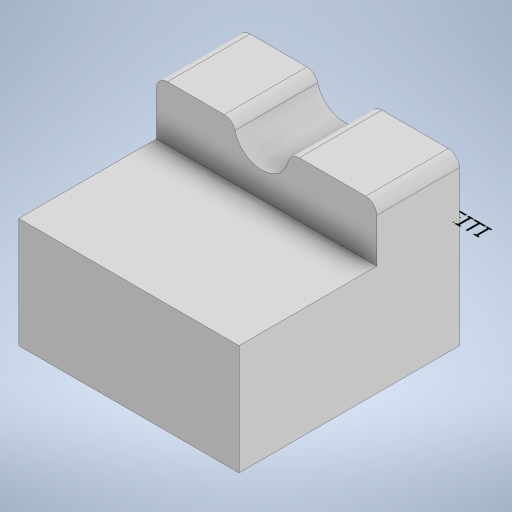
# Autodesk Inventor part: DIODA
Saved by Autodesk Inventor 2023 (Build 270158000, 158)
## iProperties
Created: 2022-12-21
Part Number: DIODA
Material: Generic
Document SubType Name: Sheet Metal
Designer: julia
Density: 1 g/cm^3
Sheet Metal Rule: Default
Appearance: Default
Author: julia
Autodesk Inventor part; units mm, degrees
ref_plane "YZ Plane" through (0, 0, 0) normal (1, 0, 0) x (0, 1, 0)
ref_plane "XZ Plane" through (0, 0, 0) normal (0, 1, 0) x (-1, 0, 0)
ref_plane "XY Plane" through (0, 0, 0) normal (0, 0, 1) x (1, 0, 0)
sketch "Sketch1" plane through (0, 0, 0) normal (0, 1, 0) x (-1, 0, 0)
  line L0 (0, 0) -> (40, 0)
  line L1 (40, 0) -> (40, 40)
  line L2 (40, 40) -> (0, 40)
  line L3 (0, 40) -> (0, 0)
  dimension "d0" = 40
  dimension "d1" = 40
  constraints: 8 end point, 2 parallel, 1 horizontal, 1 perpendicular
  measures "d0" distance of L2.end L1.end
  measures "d1" distance of L1.end L0.end
extrude "Extrusion1" add sketch "Sketch1" along normal blind 20
sketch "Sketch2" plane through (0, 20, 0) normal (0, 1, 0) x (1, 0, 0)
  line L0 (0, -40) -> (0, 0) projected
  line L1 (-40, 0) -> (-40, -40) projected
  line L2 (0, 0) -> (-40, 0)
  line L3 (-40, 0) -> (-40, -15)
  line L4 (-40, -15) -> (0, -15)
  line L5 (0, -15) -> (0, 0)
  dimension "d4" = 15
  constraints: 8 end point, 2 parallel, 1 horizontal, 1 perpendicular, 1 point on line
  measures "d4" distance of L3.end L2.end
extrude "Extrusion2" add sketch "Sketch2" along normal blind 20
sketch "Sketch3" plane through (-40, 20, 15) normal (0, 0, 1) x (1, 0, 0)
  circle A0 centre (19.125, 9.6739) radius 5
  point P0 (40, -20)
  dimension "d7" = 10
  constraints: 1 centre point
  measures "d7" diameter of A0
extrude "Extrusion3" cut sketch "Sketch3" against normal blind 20
sketch "Sketch4" plane through (-40, 20, 15) normal (0, 0, 1) x (1, 0, 0)
  line L0 (40, 20) -> (0, 20) projected
  line L1 (40, -20) -> (40, 20) projected
  line L2 (0, 20) -> (40, 20)
  line L3 (40, 20) -> (40, 10)
  line L4 (40, 10) -> (0, 10)
  line L5 (0, 10) -> (0, 20)
  dimension "d10" = 10
  constraints: 8 end point, 2 parallel, 1 horizontal, 1 perpendicular, 1 point on line
  measures "d10" distance of L2.end L3.end
extrude "Extrusion4" cut sketch "Sketch4" against normal blind 20
fillet "Fillet1" radius 2 4 edges at (-40, 30, 7.5) (-25.8644, 30, 7.5) (-15.8857, 30, 7.5) (0, 30, 7.5)
sketch "Sketch5" plane through (0, 20, 0) normal (0, 1, 0) x (1, 0, 0)
  line L0 (-4.8773, 1.27) -> (4.8773, 1.27) construction
  line L1 (4.8773, 1.27) -> (4.8773, -1.27) construction
  line L2 (4.8773, -1.27) -> (-4.8773, -1.27) construction
  line L3 (-4.8773, -1.27) -> (-4.8773, 1.27) construction
  point P0 (0, 0)
  constraints: 2 other
equation "\"BendRadius\" = Thickness"
equation "\"BendReliefWidth\" = Thickness"
equation "\"BendReliefDepth\" = 0.5 * Thickness"
equation "\"CornerReliefSize\" = 4 * Thickness"
equation "\"MinimumRemnant\" = 2 * Thickness"
equation "\"TransitionRadius\" = BendRadius"
equation "\"JacobiRadiusSize\" = BendRadius"
equation "\"GapSize\" = Thickness"
equation "\"Thickness\" = 3.048"
body "Solid1"
